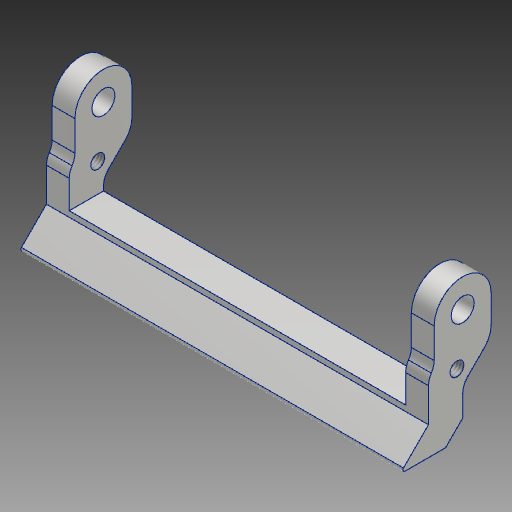
# Autodesk Inventor part: Chip Schaufel
Saved by Autodesk Inventor 2019.4 (Build 234330000, 330)
## iProperties
Part Number: Chip Schaufel
Material: Aluminium 6061
Document SubType Name: Modeling
Designer: rYan
Mass: 10.967 g
Surface Area: 30.2735 cm^2
Volume: 4.06184 cm^3
Density: 2.7 g/cm^3
Appearance: Aluminium - flach
Author: rYan
Autodesk Inventor part; units mm, degrees
ref_plane "YZ Plane" through (0, 0, 0) normal (1, 0, 0) x (0, 1, 0)
ref_plane "XZ Plane" through (0, 0, 0) normal (0, 1, 0) x (-1, 0, 0)
ref_plane "XY Plane" through (0, 0, 0) normal (0, 0, 1) x (1, 0, 0)
sketch "Skizze1" plane through (0, 0, 0) normal (1, 0, 0) x (0, 1, 0)
  line L0 (-6, 5) -> (-10.5, 0.5)
  line L1 (-10.5, 0) -> (-3, 0)
  line L2 (0, 3) -> (0, 8)
  line L3 (-10.5, 0.5) -> (-10.5, 0)
  line L4 (0, 8) -> (5, 13)
  line L5 (0, 8) -> (0, 19.5) construction
  circle A0 centre (0, 19.5) radius 0.5
  line L6 (-5, 13) -> (-5, 24.5)
  line L7 (-5, 24.5) -> (5, 24.5)
  line L8 (5, 24.5) -> (5, 13)
  line L9 (0, 3) -> (-3, 0)
  line L10 (-5, 13) -> (-6, 12)
  line L11 (-6, 12) -> (-6, 5)
  line L12 (5, 13) -> (-5, 13) construction
  point P0 (0, 0)
  dimension "d40" = 0.5
  dimension "d41" = 10.5
  dimension "d44" = 1
  dimension "d56" = 5
  dimension "d58" = 19.5
  dimension "d59" = 10
  dimension "d60" = 45
  dimension "d61" = 8
  dimension "d62" = 3
  dimension "d63" = 45
  dimension "d67" = 1
  constraints: 27 end point, 5 vertical, 2 parallel, 2 perpendicular, 2 point on line, 1 centre point, 1 coincident, 1 horizontal, 1 other
  measures "d40" distance of L0.end L1.start
  measures "d41" distance from line of L1.start L2
  measures "d44" diameter of A0
  measures "d56" distance from line of L7 L5.end
  measures "d58" distance from line of L1 L5.end
  measures "d59" distance of L6.end L7.end
  measures "d60" angle of L9 L1
  measures "d61" distance from line of L2.end L1
  measures "d62" distance of point (0, 0) L1.end
  measures "d63" angle of L0 L1
  measures "d67" distance between parallel lines of L6 L11
extrude "Extrusion1" add sketch "Skizze1" along normal mid plane 67
sketch "Skizze6" plane through (0, 0, 0) normal (0, 1, 0) x (-1, 0, 0)
  line L0 (33.5, 0.5) -> (-33.5, 0.5) projected
  line L1 (-33.5, 5) -> (-33.5, 0.5) projected
  line L2 (33.5, 0.5) -> (33.5, 5) projected
  line L3 (-29.5, 6) -> (29.5, 6)
  line L4 (29.5, 6) -> (29.5, 36)
  line L5 (29.5, 36) -> (-29.5, 36)
  line L6 (-29.5, 36) -> (-29.5, 6)
  line L7 (0, -7.1) -> (0, 42.6) projected
  line L8 (33.5, 0) -> (-33.5, 0) projected
  line L9 (-33.5, 0) -> (33.5, 0) projected
  point P0 (0, 0)
  point P1 (-33, 10)
  point P2 (33, 10)
  dimension "d45" = 4
  dimension "d46" = 30
  dimension "d50" = 6
  constraints: 8 end point, 2 parallel, 1 horizontal, 1 perpendicular, 3 other
  measures "d46" distance of L3.end L4.end
  measures "d50" distance between parallel lines of L8 L3
extrude "Extrusion4" cut sketch "Skizze6" along normal through all both and the other way through all
sketch "Skizze3" plane through (-33.5, 0, 0) normal (-1, 0, 0) x (0, 0, 1)
  line L0 (8, 0) -> (3, 0) projected
  line L1 (0, -3) -> (0, -10.5) projected
  line L2 (0.5, -10.5) -> (5, -6) projected
  line L3 (0, -10.5) -> (0, 0) construction
  line L4 (0, 8.1) -> (0, -13.6) projected
  line L5 (0, -10.5) -> (0.5, -10.5) projected
  line L6 (13, 5) -> (8, 0) projected
  line L7 (13, -5) -> (24.5, -5) projected
  line L8 (24.5, -5) -> (24.5, 5) projected
  line L9 (24.5, 5) -> (13, 5) projected
  circle A0 centre (19.5, 0) radius 0.5 projected
  line L10 (3, 0) -> (0, -3) projected
  line L11 (5, -6) -> (12, -6) projected
  line L12 (12, -6) -> (13, -5) projected
  constraints: 1 coincident
hole "Bohrung1" at (-33.5, 0, 19.5) direction (1, 0, 0) diameter 4.05 end through all
sketch "Skizze4" plane through (-33.5, 0, 0) normal (-1, 0, 0) x (0, 0, 1)
  line L0 (8, 0) -> (0, 0) projected
  line L1 (0, 8.1) -> (0, -13.6) projected
  point P0 (29, 0)
  point P1 (11, -1)
  dimension "d38" = 11
  dimension "d69" = 1
  measures "d38" distance from line of point (11, -1) L1
  measures "d69" distance from line of L0 point (11, -1)
hole "Bohrung2" at (-33.5, -1, 11) direction (1, 0, 0) diameter 2.459 end through all thread size "M3x0.5" class "6H" standard "ISO Metric profile"
fillet "Rundung1" [suppressed]
fillet "Rundung2" radius 5 4 edges at (31.5, -5, 24.5) (31.5, 5, 24.5) (-31.5, 5, 24.5) (-31.5, -5, 24.5)
fillet "Rundung5" radius 4 2 edges at (31.5, 5, 13) (-31.5, 5, 13)
fillet "Rundung7" radius 3 6 edges at (-31.5, 0, 8) (31.5, 0, 8) (31.5, -6, 12) (31.5, -5, 13) (-31.5, -6, 12) (-31.5, -5, 13)
fillet "Rundung8" radius 0.36 2 edges at (0, -10.5, 0.5) (0, -10.5, 0)
